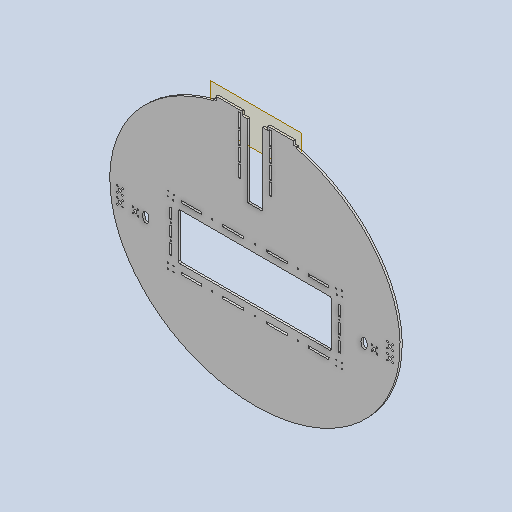
# Autodesk Inventor part: основа_лица
Saved by Autodesk Inventor 2023 (Build 270158000, 158)
## iProperties
Created: 2025-02-03
Part Number: основа_лица
Material: Типовые
Document SubType Name: Modeling
Designer: baranovaem
Density: 1 g/cm^3
Appearance: По умолчанию
Author: baranovaem
Autodesk Inventor part; units mm, degrees
ref_plane "YZ Plane" through (0, 0, 0) normal (1, 0, 0) x (0, 1, 0)
ref_plane "XZ Plane" through (0, 0, 0) normal (0, 1, 0) x (-1, 0, 0)
ref_plane "XY Plane" through (0, 0, 0) normal (0, 0, 1) x (1, 0, 0)
ref_plane "РабПлоскость1" through (0, 0, 0) normal (0, 0, 1) x (-1, 0, 0)
sketch "Эскиз2" plane through (0, 0, 0) normal (0, 0, 1) x (-1, 0, 0)
  line L0 (-80.017, -3.6447) -> (-79.9992, 0.3553)
  line L1 (79.9992, -0.3553) -> (79.9846, -3.6447)
  line L2 (79.9992, -0.3553) -> (79.9992, 5.9844)
  line L3 (-79.9992, 5.9842) -> (-79.9992, 0.3553)
  line L4 (-79.872, 29) -> (-79.9992, 29)
  ellipse E0 centre (-0.0004, 235.9801) end of major axis (-280.0004, 235.9801) minor radius 240 (79.9992, 5.9844) -> (-79.9992, 5.9842) ccw
  line L5 (79.9846, -3.6447) -> (-80.017, -3.6447)
  dimension "d80" = 240
  dimension "d46" = 9.6289
  constraints: 12 end point, 2 perpendicular, 1 horizontal, 1 point on line, 1 vertical, 4 other
  measures "d46" distance of L0.start L3.start
extrude "Выдавливание1" add sketch "Эскиз2" along normal mid plane 4
sketch "Эскиз3" plane through (0, 0, -2) normal (0, 0, -1) x (-1, 0, 0)
  line L0 (177.5, -340.9801) -> (-177.5, -340.9801)
  line L1 (-177.5, -340.9801) -> (-177.5, -190.9801)
  line L2 (-177.5, -130.9801) -> (177.5, -130.9801) construction
  line L3 (177.5, -130.9801) -> (177.5, -190.9801) construction
  line L4 (177.5, -340.9801) -> (-177.5, -130.9801) construction
  line L5 (0, 0) -> (0, -542.8198) construction
  ellipse E0 centre (-0.0004, -235.9801) end of major axis (-280.0004, -235.9801) minor radius 240 (-79.9992, -5.9842) -> (79.9992, -5.9844) ccw projected
  circle A0 centre (-162.5, -325.9801) radius 15
  line L6 (177.5, -190.9801) -> (-177.5, -190.9801)
  line L7 (177.5, -190.9801) -> (177.5, -340.9801)
  line L8 (-177.5, -190.9801) -> (-177.5, -130.9801) construction
  line L9 (177.5, -265.9801) -> (-177.5, -265.9801) construction
  circle A1 centre (-162.5, -205.9801) radius 15
  line L10 (144.5, -310.9801) -> (-144.5, -310.9801)
  line L11 (144.5, -220.9801) -> (-144.5, -220.9801)
  line L12 (147.5, -307.9801) -> (147.5, -223.9801)
  line L13 (-147.5, -307.9801) -> (-147.5, -223.9801)
  arc A2 (144.5, -310.9801) -> (147.5, -307.9801) centre (144.5, -307.9801) ccw
  arc A3 (147.5, -223.9801) -> (144.5, -220.9801) centre (144.5, -223.9801) ccw
  arc A4 (-144.5, -220.9801) -> (-147.5, -223.9801) centre (-144.5, -223.9801) ccw
  arc A5 (-147.5, -307.9801) -> (-144.5, -310.9801) centre (-144.5, -307.9801) ccw
  circle A6 centre (157.0187, -331.0005) radius 1.25 projected
  circle A7 centre (168.0186, -330.9595) radius 1.25 projected
  circle A8 centre (167.9813, -320.9596) radius 1.25 projected
  circle A9 centre (156.9814, -321.0006) radius 1.25 projected
  circle A10 centre (168.6444, -210.1629) radius 1.25 projected
  circle A11 centre (157.7523, -211.6992) radius 1.25 projected
  circle A12 centre (167.2477, -200.2609) radius 1.25 projected
  circle A13 centre (156.3556, -201.7972) radius 1.25 projected
  line L14 (-177.5, -340.9801) -> (177.5, -130.9801) construction
  circle A14 centre (-157.0187, -331.0005) radius 1.25
  circle A15 centre (-168.0186, -330.9595) radius 1.25
  circle A16 centre (-167.9813, -320.9596) radius 1.25
  circle A17 centre (-156.9814, -321.0006) radius 1.25
  circle A18 centre (-168.6444, -210.1629) radius 1.25
  circle A19 centre (-157.7523, -211.6992) radius 1.25
  circle A20 centre (-167.2477, -200.2609) radius 1.25
  circle A21 centre (-156.3556, -201.7972) radius 1.25
  point P0 (0, -235.9801)
  point P1 (177.5, -310.9801)
  point P2 (-177.5, -310.9801)
  point P3 (177.5, -220.9801)
  point P4 (-177.5, -220.9801)
  point P5 (147.5, -340.9801)
  point P6 (147.5, -190.9801)
  point P7 (-147.5, -340.9801)
  point P8 (-147.5, -190.9801)
  dimension "d4" = 355
  dimension "d5" = 210
  dimension "d6" = 0
  dimension "d8" = 60
  dimension "d9" = 3
  constraints: 30 end point, 17 point on line, 14 centre point, 9 symmetric about line, 9 tangent, 8 point on circle, 6 parallel, 6 perpendicular, 3 equal radius, 3 midpoint, 2 vertical, 1 horizontal, 10 other
  measures "d4" distance of L0.start L0.end
  measures "d5" distance of L0.end L2.start
  measures "d6" vertical distance of point (0, -235.98) point (0, -235.98)
  measures "d8" distance between parallel lines of L2 L6
  measures "d9" radius of A2
extrude "Выдавливание2" cut sketch "Эскиз3" against normal blind 4 contours L10 A5 L13 A4 L11 A3 L12 A2 | A6 | A7 | A8 | A9 | A10 | A11 | A12 | A13 | A14 | A15 | A16 | A17 | A18 | A19 | A20 | A21
sketch "Эскиз4" plane through (0, 0, 2) normal (0, 0, 1) x (1, 0, 0)
  circle A0 centre (-162.5, -205.9801) radius 15 projected
  circle A1 centre (-162.5, -325.9801) radius 15 projected
  circle A2 centre (162.5, -205.9801) radius 15 projected
  circle A3 centre (162.5, -325.9801) radius 15 projected
  line L0 (164.5, -225.9801) -> (160.5, -225.9801)
  line L1 (160.5, -225.9801) -> (160.5, -305.9801)
  line L2 (160.5, -305.9801) -> (164.5, -305.9801)
  line L3 (164.5, -305.9801) -> (164.5, -225.9801)
  line L4 (-144.5, -220.9801) -> (144.5, -220.9801) projected
  line L5 (142.5, -207.9801) -> (-142.5, -207.9801)
  line L6 (-142.5, -207.9801) -> (-142.5, -203.9801)
  line L7 (-142.5, -203.9801) -> (142.5, -203.9801)
  line L8 (142.5, -203.9801) -> (142.5, -207.9801)
  line L9 (102.5, -203.9801) -> (102.5, -207.9801)
  line L10 (62.5, -203.9801) -> (62.5, -207.9801)
  line L11 (22.5, -203.9801) -> (22.5, -207.9801)
  line L12 (-102.5, -203.9801) -> (-102.5, -207.9801)
  line L13 (-62.5, -203.9801) -> (-62.5, -207.9801)
  line L14 (-22.5, -203.9801) -> (-22.5, -207.9801)
  line L15 (102.5, -204.5415) -> (142.5, -203.9801) construction
  line L16 (162.5, -205.9801) -> (102.5, -205.9801) construction
  line L17 (142.5, -207.9801) -> (102.5, -207.4187) construction
  line L18 (62.5, -206.8572) -> (22.5, -206.2958) construction
  line L19 (62.5, -205.9801) -> (22.5, -205.9801) construction
  line L20 (22.5, -205.6643) -> (62.5, -205.1029) construction
  line L21 (-22.5, -205.6643) -> (-62.5, -205.1029) construction
  line L22 (-102.5, -204.5415) -> (-142.5, -203.9801) construction
  line L23 (-22.5, -205.9801) -> (-62.5, -205.9801) construction
  line L24 (-102.5, -205.9801) -> (-162.5, -205.9801) construction
  line L25 (-142.5, -207.9801) -> (-102.5, -207.4187) construction
  line L26 (-62.5, -206.8572) -> (-22.5, -206.2958) construction
  line L27 (62.5, -207.9801) -> (102.5, -203.9801) construction
  circle A4 centre (82.5, -205.9801) radius 1.45
  line L28 (-22.5, -207.9801) -> (22.5, -203.9801) construction
  circle A5 centre (0, -205.9801) radius 1.45
  circle A6 centre (-82.5, -205.9801) radius 1.45
  line L29 (-62.5, -203.9801) -> (-102.5, -207.9801) construction
  line L30 (164.5, -285.9801) -> (160.5, -285.9801)
  line L31 (164.5, -245.9801) -> (160.5, -245.9801)
  line L32 (164.5, -255.9801) -> (160.5, -255.9801)
  line L33 (164.5, -275.9801) -> (160.5, -275.9801)
  line L34 (163.5, -285.9801) -> (164.5, -305.9801) construction
  line L35 (162.5, -325.9801) -> (162.5, -285.9801) construction
  line L36 (161.5, -285.9801) -> (160.5, -305.9801) construction
  line L37 (164.5, -225.9801) -> (163.5, -245.9801) construction
  line L38 (163, -255.9801) -> (162, -275.9801) construction
  line L39 (162.5, -275.9801) -> (162.5, -255.9801) construction
  line L40 (162.5, -245.9801) -> (162.5, -205.9801) construction
  line L41 (160.5, -225.9801) -> (161.5, -245.9801) construction
  line L42 (162, -255.9801) -> (163, -275.9801) construction
  line L43 (164.5, -245.9801) -> (160.5, -255.9801) construction
  line L44 (160.5, -275.9801) -> (164.5, -285.9801) construction
  circle A7 centre (162.5, -280.9801) radius 1.45
  circle A8 centre (162.5, -250.9801) radius 1.45
  line L45 (0, -146) -> (0, -429) construction
  line L46 (-164.5, -225.9801) -> (-160.5, -225.9801)
  line L47 (-160.5, -225.9801) -> (-160.5, -305.9801)
  line L48 (-160.5, -305.9801) -> (-164.5, -305.9801)
  line L49 (-164.5, -305.9801) -> (-164.5, -225.9801)
  line L50 (-164.5, -285.9801) -> (-160.5, -285.9801)
  line L51 (-164.5, -245.9801) -> (-160.5, -245.9801)
  line L52 (-164.5, -255.9801) -> (-160.5, -255.9801)
  line L53 (-164.5, -275.9801) -> (-160.5, -275.9801)
  line L54 (-163.5, -285.9801) -> (-164.5, -305.9801) construction
  line L55 (-162.5, -325.9801) -> (-162.5, -285.9801) construction
  line L56 (-161.5, -285.9801) -> (-160.5, -305.9801) construction
  line L57 (-164.5, -225.9801) -> (-163.5, -245.9801) construction
  line L58 (-163, -255.9801) -> (-162, -275.9801) construction
  line L59 (-162.5, -275.9801) -> (-162.5, -255.9801) construction
  line L60 (-162.5, -245.9801) -> (-162.5, -205.9801) construction
  line L61 (-160.5, -225.9801) -> (-161.5, -245.9801) construction
  line L62 (-162, -255.9801) -> (-163, -275.9801) construction
  line L63 (-164.5, -245.9801) -> (-160.5, -255.9801) construction
  line L64 (-160.5, -275.9801) -> (-164.5, -285.9801) construction
  circle A9 centre (-162.5, -280.9801) radius 1.45
  circle A10 centre (-162.5, -250.9801) radius 1.45
  line L65 (-162.5, -265.9801) -> (162.5, -265.9801) construction
  line L66 (142.5, -323.9801) -> (-142.5, -323.9801)
  line L67 (-142.5, -323.9801) -> (-142.5, -327.9801)
  line L68 (-142.5, -327.9801) -> (142.5, -327.9801)
  line L69 (142.5, -327.9801) -> (142.5, -323.9801)
  line L70 (102.5, -327.9801) -> (102.5, -323.9801)
  line L71 (62.5, -327.9801) -> (62.5, -323.9801)
  line L72 (22.5, -327.9801) -> (22.5, -323.9801)
  line L73 (-102.5, -327.9801) -> (-102.5, -323.9801)
  line L74 (-62.5, -327.9801) -> (-62.5, -323.9801)
  line L75 (-22.5, -327.9801) -> (-22.5, -323.9801)
  line L76 (102.5, -327.4187) -> (142.5, -327.9801) construction
  line L77 (142.5, -323.9801) -> (102.5, -324.5415) construction
  line L78 (62.5, -325.1029) -> (22.5, -325.6643) construction
  line L79 (62.5, -325.9801) -> (22.5, -325.9801) construction
  line L80 (22.5, -326.2958) -> (62.5, -326.8572) construction
  line L81 (-22.5, -326.2958) -> (-62.5, -326.8572) construction
  line L82 (-102.5, -327.4187) -> (-142.5, -327.9801) construction
  line L83 (-22.5, -325.9801) -> (-62.5, -325.9801) construction
  line L84 (-142.5, -323.9801) -> (-102.5, -324.5415) construction
  line L85 (-62.5, -325.1029) -> (-22.5, -325.6643) construction
  line L86 (62.5, -323.9801) -> (102.5, -327.9801) construction
  circle A11 centre (82.5, -325.9801) radius 1.45
  line L87 (-22.5, -323.9801) -> (22.5, -327.9801) construction
  circle A12 centre (0, -325.9801) radius 1.45
  circle A13 centre (-82.5, -325.9801) radius 1.45
  line L88 (-62.5, -327.9801) -> (-102.5, -323.9801) construction
  point P0 (0, 0)
  point P1 (147.6339, -207.9801)
  point P2 (147.6339, -203.9801)
  point P3 (142.5, -205.9801)
  point P4 (-82.5, -205.9801)
  point P5 (144.5, -310.9801)
  point P6 (-102.5, -325.9801)
  point P7 (102.5, -325.9801)
  point P8 (142.5, -325.9801)
  point P9 (0, -385.9601)
  dimension "d16" = 4
  dimension "d17" = 80
  dimension "d18" = 285
  dimension "d19" = 4
  dimension "d27" = 40
  dimension "d28" = 40
  dimension "d29" = 40
  dimension "d30" = 40
  dimension "d31" = 40
  dimension "d32" = 40
  dimension "d33" = 2.9
  dimension "d34" = 2.9
  dimension "d35" = 2.9
  dimension "d36" = 20
  dimension "d37" = 20
  dimension "d38" = 10
  dimension "d39" = 10
  dimension "d40" = 2.9
  dimension "d41" = 2.9
  constraints: 176 end point, 80 point on line, 69 symmetric about line, 39 midpoint, 13 perpendicular, 10 centre point, 8 parallel, 4 vertical, 2 coincident, 2 horizontal, 5 other
  measures "d16" distance of L2.end L1.end
  measures "d17" distance of L1.end L0.end
  measures "d18" distance of L6.end L7.end
  measures "d19" distance of L5.end L6.end
  measures "d27" horizontal distance of L24.start L6.end
  measures "d28" distance of L24.start L23.end
  measures "d29" distance from line of L23.end L14
  measures "d30" distance of L16.end point (142.5, -205.98)
  measures "d31" horizontal distance of L10.end L16.end
  measures "d32" distance between parallel lines of L10 L11
  measures "d33" diameter of A4
  measures "d34" diameter of A5
  measures "d35" diameter of A6
  measures "d36" distance between parallel lines of L0 L31
  measures "d37" distance between parallel lines of L30 L2
  measures "d38" distance of L35.end L39.start
  measures "d39" distance of L40.start L39.end
  measures "d40" diameter of A7
  measures "d41" diameter of A8
extrude "Выдавливание3" cut sketch "Эскиз4" against normal blind 4 contours L3 L31 L1 L0 | L3 L33 L1 L32 | L3 L2 L1 L30 | L5 L9 L7 L8 | L5 L11 L7 L10 | L5 L13 L7 L14 | L5 L6 L7 L12 | A4 | A5 | A6 | A7 | A8 | L46 L47 L51 L49 | L52 L47 L53 L49 | L50 L47 L48 L49 | A9 | A10 | L69 L68 L70 L66 | L71 L68 L72 L66 | L75 L68 L74 L66 | L73 L68 L67 L66 | A11 | A12 | A13
sketch "Эскиз5" plane through (0, 0, -2) normal (0, 0, -1) x (-1, 0, 0)
  line L0 (75, -3.6447) -> (-75, -3.6447)
  line L1 (-75, -3.6447) -> (-75, 3.6447)
  line L2 (-75, 3.6447) -> (75, 3.6447)
  line L3 (75, 3.6447) -> (75, -3.6447)
  line L4 (75, -3.6447) -> (-75, 3.6447) construction
  line L5 (-75, -3.6447) -> (75, 3.6447) construction
  line L6 (25, -3.6447) -> (25, 3.6447)
  line L7 (-25, -3.6447) -> (-25, 3.6447)
  line L8 (-75, -3.6447) -> (-80.017, -3.6447)
  line L9 (-79.9992, -0.3553) -> (-80.017, 3.6447) projected
  line L10 (-80.017, 3.6447) -> (-80.017, -3.6447)
  line L11 (-79.9992, -5.9842) -> (-79.9992, -0.3553) projected
  line L12 (75, 3.6447) -> (91, 3.6447)
  line L13 (91, 3.6447) -> (91, -3.6447)
  line L14 (91, -3.6447) -> (75, -3.6447)
  line L15 (75, -3.6447) -> (75, 3.6447)
  line L16 (-80.017, 3.6447) -> (79.9846, 3.6447) projected
  line L17 (-75, 3.6447) -> (-80.017, 3.6447)
  point P0 (0, 0)
  point P1 (-79.9992, -3.6447)
  point P2 (25, 3.6447)
  dimension "d22" = 150
  dimension "d23" = 50
  dimension "d24" = 50
  constraints: 30 end point, 4 horizontal, 4 parallel, 4 perpendicular, 3 point on line, 2 midpoint, 1 vertical, 1 other
  measures "d22" distance of L1.end L2.end
  measures "d23" distance between parallel lines of L1 L7
  measures "d24" distance between parallel lines of L6 L3
extrude "Выдавливание4" cut sketch "Эскиз5" against normal blind 4 contours L3 L12 L13 L14 | L0 L7 L2 L6 | L8 L11 L9 L16 L1 | L8 L10 L9 L11
sketch "Эскиз6" plane through (0, 0, 2) normal (0, 0, 1) x (1, 0, 0)
  line L0 (14, -143.6447) -> (-14, -143.6447)
  line L1 (-14, -143.6447) -> (-14, -3.6447)
  line L2 (-14, -3.6447) -> (14, -3.6447)
  line L3 (14, -3.6447) -> (14, -143.6447)
  line L4 (14, -143.6447) -> (-14, -3.6447) construction
  line L5 (-14, -143.6447) -> (14, -3.6447) construction
  line L6 (25, -3.6447) -> (-25, -3.6447) projected
  point P0 (0, 0)
  point P1 (0, -73.6447)
  point P2 (0, -3.6447)
  dimension "d42" = 28
  dimension "d43" = 140
  constraints: 12 end point, 4 midpoint, 2 parallel, 1 horizontal, 1 perpendicular
  measures "d42" distance of L1.end L2.end
  measures "d43" distance of L0.end L1.end
extrude "Выдавливание5" cut sketch "Эскиз6" against normal blind 4
sketch "Эскиз7" plane through (0, 0, -2) normal (0, 0, -1) x (-1, 0, 0)
  line L0 (-31.408, -0.3553) -> (-28.408, -0.3553)
  line L1 (-28.408, -0.3553) -> (-28.408, -28.3553)
  line L2 (-28.408, -31.3553) -> (-28.408, -56.3553)
  line L3 (-31.408, -59.3553) -> (-28.408, -59.3553)
  line L4 (-31.408, -111.1218) -> (-31.408, -87.3553)
  line L5 (-31.408, -87.3553) -> (-28.408, -87.3553)
  line L6 (-28.408, -84.3553) -> (-31.408, -84.3553)
  line L7 (-31.408, -84.3553) -> (-31.408, -59.3553)
  line L8 (-28.408, -111.1218) -> (-31.408, -111.1218)
  line L9 (-31.408, -3.3553) -> (-31.408, -0.3553)
  line L10 (-31.408, -28.3553) -> (-31.408, -3.3553)
  line L11 (-31.408, -56.3553) -> (-31.408, -31.3553)
  line L12 (-28.408, -28.3553) -> (-31.408, -28.3553)
  line L13 (-31.408, -31.3553) -> (-28.408, -31.3553)
  line L14 (-28.408, -56.3553) -> (-31.408, -56.3553)
  line L15 (-28.408, -59.3553) -> (-28.408, -84.3553)
  line L16 (-28.408, -87.3553) -> (-28.408, -111.1218)
  point P0 (0, 0)
  constraints: 34 end point
extrude "Выдавливание6" cut sketch "Эскиз7" against normal blind 4
sketch "Эскиз8" plane through (0, 0, 2) normal (0, 0, 1) x (1, 0, 0)
  line L0 (-31.408, -0.3553) -> (-28.408, -0.3553)
  line L1 (-28.408, -0.3553) -> (-28.408, -28.3553)
  line L2 (-28.408, -31.3553) -> (-28.408, -56.3553)
  line L3 (-31.408, -59.3553) -> (-28.408, -59.3553)
  line L4 (-31.408, -111.1218) -> (-31.408, -87.3553)
  line L5 (-31.408, -87.3553) -> (-28.408, -87.3553)
  line L6 (-28.408, -84.3553) -> (-31.408, -84.3553)
  line L7 (-31.408, -84.3553) -> (-31.408, -59.3553)
  line L8 (-28.408, -111.1218) -> (-31.408, -111.1218)
  line L9 (-31.408, -3.3553) -> (-31.408, -0.3553)
  line L10 (-31.408, -28.3553) -> (-31.408, -3.3553)
  line L11 (-31.408, -56.3553) -> (-31.408, -31.3553)
  line L12 (-28.408, -28.3553) -> (-31.408, -28.3553)
  line L13 (-31.408, -31.3553) -> (-28.408, -31.3553)
  line L14 (-28.408, -56.3553) -> (-31.408, -56.3553)
  line L15 (-28.408, -59.3553) -> (-28.408, -84.3553)
  line L16 (-28.408, -87.3553) -> (-28.408, -111.1218)
  point P0 (0, 0)
  constraints: 34 end point
extrude "Выдавливание7" cut sketch "Эскиз8" against normal blind 4
sketch "Эскиз9" plane through (0, 0, -2) normal (0, 0, -1) x (-1, 0, 0)
  line L0 (-160.5, -255.9801) -> (-260.5, -255.9801) construction
  line L1 (-260.5, -255.9801) -> (-260.5, -277) construction
  line L2 (-260.5, -277) -> (-160.5, -277) construction
  line L3 (-160.5, -277) -> (-160.5, -255.9801) construction
  circle A0 centre (217.2499, 89.3506) radius 1.6806
  circle A1 centre (212.1896, 94.5548) radius 3.0463
  circle A2 centre (217.3783, 99.3507) radius 1.6805
  circle A3 centre (206.8799, 99.3342) radius 1.6809
  circle A4 centre (206.8954, 89.3342) radius 1.6807
  circle A5 centre (217.2499, 89.3506) radius 1.6806
  circle A6 centre (212.1896, 94.5548) radius 3.0463
  circle A7 centre (217.3783, 99.3507) radius 1.6805
  circle A8 centre (206.8799, 99.3342) radius 1.6809
  circle A9 centre (206.8954, 89.3342) radius 1.6807
  circle A10 centre (-260.5, -266.49) radius 3
  line L4 (-255.5, -271.74) -> (-265.5, -271.74) construction
  line L5 (-265.5, -271.74) -> (-265.5, -261.24) construction
  line L6 (-265.5, -261.24) -> (-255.5, -261.24) construction
  line L7 (-255.5, -261.24) -> (-255.5, -271.74) construction
  line L8 (-255.5, -271.74) -> (-265.5, -261.24) construction
  line L9 (-265.5, -271.74) -> (-255.5, -261.24) construction
  circle A11 centre (-265.5, -271.74) radius 1.65
  circle A12 centre (-265.5, -261.24) radius 1.65
  circle A13 centre (-255.5, -261.24) radius 1.65
  circle A14 centre (-255.5, -271.74) radius 1.65
  circle A15 centre (-230.5, -266.49) radius 3
  line L10 (-225.5, -271.74) -> (-235.5, -271.74) construction
  line L11 (-235.5, -271.74) -> (-235.5, -261.24) construction
  line L12 (-235.5, -261.24) -> (-225.5, -261.24) construction
  line L13 (-225.5, -261.24) -> (-225.5, -271.74) construction
  line L14 (-225.5, -271.74) -> (-235.5, -261.24) construction
  line L15 (-235.5, -271.74) -> (-225.5, -261.24) construction
  circle A16 centre (-235.5, -271.74) radius 1.65
  circle A17 centre (-235.5, -261.24) radius 1.65
  circle A18 centre (-225.5, -261.24) radius 1.65
  circle A19 centre (-225.5, -271.74) radius 1.65
  circle A20 centre (-260.5, -246.49) radius 3
  line L16 (-255.5, -251.74) -> (-265.5, -251.74) construction
  line L17 (-265.5, -251.74) -> (-265.5, -241.24) construction
  line L18 (-265.5, -241.24) -> (-255.5, -241.24) construction
  line L19 (-255.5, -241.24) -> (-255.5, -251.74) construction
  line L20 (-255.5, -251.74) -> (-265.5, -241.24) construction
  line L21 (-265.5, -251.74) -> (-255.5, -241.24) construction
  circle A21 centre (-265.5, -251.74) radius 1.65
  circle A22 centre (-265.5, -241.24) radius 1.65
  circle A23 centre (-255.5, -241.24) radius 1.65
  circle A24 centre (-255.5, -251.74) radius 1.65
  line L22 (0, -160) -> (0, -379) construction
  line L23 (160.5, -255.9801) -> (260.5, -255.9801) construction
  line L24 (260.5, -255.9801) -> (260.5, -277) construction
  line L25 (260.5, -277) -> (160.5, -277) construction
  circle A25 centre (260.5, -266.49) radius 3
  line L26 (255.5, -271.74) -> (265.5, -271.74) construction
  line L27 (265.5, -271.74) -> (265.5, -261.24) construction
  line L28 (265.5, -261.24) -> (255.5, -261.24) construction
  line L29 (255.5, -261.24) -> (255.5, -271.74) construction
  line L30 (255.5, -271.74) -> (265.5, -261.24) construction
  line L31 (265.5, -271.74) -> (255.5, -261.24) construction
  circle A26 centre (265.5, -271.74) radius 1.65
  circle A27 centre (265.5, -261.24) radius 1.65
  circle A28 centre (255.5, -261.24) radius 1.65
  circle A29 centre (255.5, -271.74) radius 1.65
  line L32 (225.5, -261.24) -> (225.5, -271.74) construction
  circle A30 centre (230.5, -266.49) radius 3
  line L33 (235.5, -261.24) -> (225.5, -261.24) construction
  line L34 (225.5, -271.74) -> (235.5, -261.24) construction
  line L35 (235.5, -271.74) -> (225.5, -261.24) construction
  line L36 (225.5, -271.74) -> (235.5, -271.74) construction
  line L37 (235.5, -271.74) -> (235.5, -261.24) construction
  circle A31 centre (235.5, -271.74) radius 1.65
  circle A32 centre (235.5, -261.24) radius 1.65
  circle A33 centre (225.5, -261.24) radius 1.65
  circle A34 centre (225.5, -271.74) radius 1.65
  line L38 (255.5, -241.24) -> (255.5, -251.74) construction
  circle A35 centre (260.5, -246.49) radius 3
  line L39 (265.5, -241.24) -> (255.5, -241.24) construction
  line L40 (255.5, -251.74) -> (265.5, -241.24) construction
  line L41 (265.5, -251.74) -> (255.5, -241.24) construction
  line L42 (255.5, -251.74) -> (265.5, -251.74) construction
  line L43 (265.5, -251.74) -> (265.5, -241.24) construction
  circle A36 centre (265.5, -251.74) radius 1.65
  circle A37 centre (265.5, -241.24) radius 1.65
  circle A38 centre (255.5, -241.24) radius 1.65
  circle A39 centre (255.5, -251.74) radius 1.65
  ellipse E0 centre (210.5, -266.49) end of major axis (210.6997, -256.492) minor radius 6
  ellipse E1 centre (-210.5, -266.49) end of major axis (-210.5, -256.49) minor radius 6
  point P0 (0, 0)
  point P1 (230.5, -266.49)
  dimension "d75" = 10
  dimension "d77" = 6
  dimension "d51" = 100
  dimension "d52" = 6
  dimension "d53" = 10
  dimension "d54" = 10.5
  dimension "d55" = 3.3
  dimension "d56" = 3.3
  dimension "d57" = 3.3
  dimension "d58" = 6
  dimension "d59" = 10
  dimension "d60" = 10.5
  dimension "d61" = 3.3
  dimension "d62" = 3.3
  dimension "d63" = 3.3
  dimension "d64" = 6
  dimension "d65" = 10
  dimension "d66" = 10.5
  dimension "d67" = 3.3
  dimension "d68" = 3.3
  dimension "d69" = 3.3
  dimension "d70" = 30
  dimension "d71" = 20
  dimension "d72" = 20
  dimension "d73" = 10
  dimension "d74" = 20
  dimension "d76" = 6
  constraints: 88 end point, 41 centre point, 31 symmetric about line, 24 coincident, 8 midpoint, 8 parallel, 4 horizontal, 4 perpendicular, 1 vertical, 17 other
  measures "d51" distance of L2.end L1.end
  measures "d52" diameter of A10
  measures "d53" distance of L5.end L6.end
  measures "d54" distance of L6.end L4.start
  measures "d55" diameter of A11
  measures "d56" diameter of A12
  measures "d57" diameter of A14
  measures "d58" diameter of A15
  measures "d59" distance of L12.start L13.start
  measures "d60" distance of L13.start L13.end
  measures "d61" diameter of A16
  measures "d62" diameter of A17
  measures "d63" diameter of A19
  measures "d64" diameter of A20
  measures "d65" distance of L18.start L19.start
  measures "d66" distance of L19.start L19.end
  measures "d67" diameter of A21
  measures "d68" diameter of A22
  measures "d69" diameter of A24
  measures "d70" distance of A15.centre A10.centre
  measures "d71" distance of A20.centre A10.centre
  measures "d72" distance of E0.centre point (230.5, -266.49)
  measures "d74" distance of point (-210.5, -266.49) A15.centre
extrude "Выдавливание8" cut sketch "Эскиз9" against normal blind 4 contours A10 | A11 | A12 | A13 | A14 | A15 | A16 | A17 | A18 | A19 | A20 | A21 | A22 | A23 | A24 | A25 | A26 | A27 | A28 | A29 | A30 | A31 | A32 | A33 | A34 | A35 | A36 | A37 | A38 | A39 | E0 | E1
